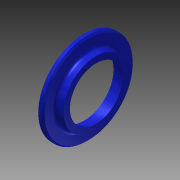
# Autodesk Inventor part: Big Bearing Cover
Saved by Autodesk Inventor 2014 (Build 180170000, 170)
## iProperties
Created: 2015-02-07
Part Number: Big Bearing Cover
Material: Generic
Document SubType Name: Modeling
Designer: Spooner
Density: 1 g/cm^3
Appearance: Blue - Wall Paint - Glossy
Author: Spooner
Autodesk Inventor part; units mm, degrees
ref_plane "YZ Plane" through (0, 0, 0) normal (1, 0, 0) x (0, 1, 0)
ref_plane "XZ Plane" through (0, 0, 0) normal (0, 1, 0) x (-1, 0, 0)
sketch "Sketch1" plane through (0, 0, 0) normal (0, 0, 1) x (1, 0, 0)
  line L0 (0, -23.495) -> (13.97, -23.495)
  line L1 (0, 23.495) -> (0, -23.495) projected
  line L2 (13.97, -23.495) -> (13.97, 23.495) projected
  line L3 (2.54, -27.305) -> (-12.065, -27.305) projected
  line L4 (26.035, -27.305) -> (11.43, -27.305) projected
  line L5 (2.54, -31.115) -> (2.54, -27.305) projected
  line L6 (11.43, -27.305) -> (11.43, -31.115) projected
  line L7 (0, -31.115) -> (2.54, -31.115) projected
  line L8 (11.43, -31.115) -> (13.97, -31.115) projected
  line L9 (3.175, -36.449) -> (10.795, -36.449)
  line L10 (10.795, -36.449) -> (10.795, -28.7565)
  line L11 (3.175, -36.449) -> (3.175, -28.7565)
  line L12 (-2.794, -26.035) -> (0.4535, -26.035)
  line L13 (-0.254, -23.749) -> (14.224, -23.749)
  line L14 (14.224, -23.749) -> (14.224, -20.955)
  line L15 (14.224, -20.955) -> (16.764, -20.955)
  line L16 (16.764, -20.955) -> (16.764, -26.035)
  line L17 (16.764, -26.035) -> (13.5165, -26.035)
  arc A0 (3.175, -28.7565) -> (0.4535, -26.035) centre (0.4535, -28.7565) ccw
  arc A1 (13.5165, -26.035) -> (10.795, -28.7565) centre (13.5165, -28.7565) ccw
  line L18 (-19.685, 0) -> (33.655, 0) projected
  line L19 (-2.794, -26.035) -> (-2.794, -20.955)
  line L20 (-2.794, -20.955) -> (-0.254, -20.955)
  line L21 (-0.254, -20.955) -> (-0.254, -23.749)
  point P0 (0, 0)
  dimension "d0" = 0.635
  dimension "d1" = 0.635
  dimension "d2" = 7.62
  dimension "d3" = 0.254
  dimension "d4" = 0.254
  dimension "d5" = 2.54
  dimension "d6" = 2.54
  dimension "d7" = 1.27
  dimension "d9" = 12.7
  dimension "d10" = 2.5418
  constraints: 26 end point, 6 parallel, 4 perpendicular, 4 point on circle, 4 tangent, 3 equal length, 2 centre point, 1 equal radius, 1 horizontal, 1 horizontal alignment, 1 vertical, 2 other
  measures "d0" distance between parallel lines of L11 L5
  measures "d1" distance between parallel lines of L6 L10
  measures "d2" distance of L9.start L9.end
  measures "d3" distance between parallel lines of L0 L13
  measures "d4" distance between parallel lines of L14 L2
  measures "d5" distance of L14.end L15.end
  measures "d6" distance between parallel lines of L0 L15
  measures "d7" distance between parallel lines of L4 L17
  measures "d9" distance between parallel lines of L13 L9
  measures "d10" distance of A0.centre L3.start
revolve "Revolution1" add sketch "Sketch1" angle 360 about axis through (-10, 0, 0) along (1, 0, 0) contours L11 A0 L12 L19 L20 L21 L13 L14 L15 L16 L17 A1 L10 L9
chamfer "Chamfer1" distance 1.27 angle 45 2 edges at (10.795, 36.449, 0) (3.175, 36.449, 0)
ref_plane "Work Plane1" through (6.985, 0, 0) normal (1, 0, 0) x (0, 0, -1)
sketch "Sketch2" plane through (6.985, 0, 0) normal (1, 0, 0) x (0, 0, -1)
  line L0 (58.906, -57.765) -> (-58.906, -57.765)
  line L1 (-58.906, -57.765) -> (-58.906, 57.765)
  line L2 (-58.906, 57.765) -> (58.906, 57.765)
  line L3 (58.906, 57.765) -> (58.906, -57.765)
  line L4 (58.906, -57.765) -> (-58.906, 57.765) construction
  line L5 (-58.906, -57.765) -> (58.906, 57.765) construction
  point P0 (0, 0)
  constraints: 12 end point, 2 midpoint, 2 parallel, 1 horizontal, 1 perpendicular
extrude "Extrusion1" cut sketch "Sketch2" against normal through all
chamfer "Chamfer2" distance 1.27 angle 45 1 edges at (14.224, 23.749, 0)
equation "\"d1\" = d0"
equation "\"d4\" = d3"
body "Solid1"
